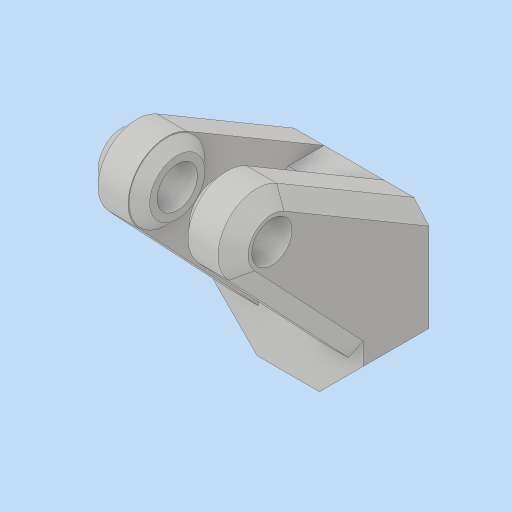
# Autodesk Inventor part: kladka-midwheel_wBearing-atTprofile
Saved by Autodesk Inventor 2024 (Build 280153000, 153)
## iProperties
Created: 2023-04-19
Part Number: kladka-midwheel_wBearing-atTprofile
Material: Generic
Document SubType Name: Modeling
Designer: Karbosch
Density: 1 g/cm^3
Appearance: Default
Mass: 2.94353 g
Surface Area: 19.3732 cm^2
Volume: 2.94353 cm^3
Author: Karbosch
Autodesk Inventor part; units mm, degrees
ref_plane "YZ Plane" through (0, 0, 0) normal (1, 0, 0) x (0, 1, 0)
ref_plane "XZ Plane" through (0, 0, 0) normal (0, 1, 0) x (-1, 0, 0)
ref_plane "XY Plane" through (0, 0, 0) normal (0, 0, 1) x (1, 0, 0)
sketch "Sketch1" plane through (0, 0, 0) normal (0, 0, 1) x (1, 0, 0)
  circle A0 centre (0, 0) radius 2.15
  line L0 (3.3137, 8) -> (8, 3.3137)
  line L1 (8, 3.3137) -> (8, -3.3137)
  line L2 (8, -3.3137) -> (3.3137, -8)
  line L3 (3.3137, -8) -> (-3.3137, -8)
  line L4 (-3.3137, -8) -> (-8, -3.3137)
  line L5 (-8, -3.3137) -> (-8, 3.3137)
  line L6 (-8, 3.3137) -> (-3.3137, 8)
  line L7 (-3.3137, 8) -> (3.3137, 8)
  dimension "d0" = 4.3
  dimension "d1" = 16
  constraints: 16 end point, 2 coincident, 1 centre point, 1 horizontal, 17 other
  measures "d0" diameter of A0
  measures "d1" distance between parallel lines of L3 L7
extrude "Extrusion1" add sketch "Sketch1" along normal blind 7
sketch "Sketch2" plane through (8, -3.3137, 0) normal (1, 0, 0) x (0, 0, -1)
  line L0 (0, 0) -> (-7, 0) projected
  line L1 (0, 6.6274) -> (0, 0) projected
  line L2 (0, 11.3137) -> (0, 6.6274) projected
  circle A0 centre (-16.7618, 16.384) radius 2.15
  circle A1 centre (-16.7618, 16.384) radius 4.15
  line L3 (0, 11.3137) -> (-7, 11.3137) projected
  line L4 (0, 11.3137) -> (-14.6531, 19.9583)
  line L5 (-7, 0) -> (-7, -4.6863) projected
  line L6 (-7, 0) -> (-19.7793, 13.5349)
  line L7 (-7, 1.1637) -> (-7, 5.4637) projected
  line L8 (-7, 3.3137) -> (-11, 3.3137)
  line L9 (-11, 3.3137) -> (-11, 7.0137)
  circle A2 centre (-16.7618, 16.384) radius 11
  point P0 (0, 3.3137)
  dimension "d4" = 4.3
  dimension "d6" = 2
  dimension "d17" = 4
  dimension "d18" = 3.7
  dimension "d19" = 22
  constraints: 8 end point, 4 point on circle, 3 centre point, 2 coincident, 2 tangent, 1 horizontal, 1 midpoint, 1 vertical
  measures "d4" diameter of A0
  measures "d6" radial gap between concentric circles of A1 A0
  measures "d17" distance of L8.start L8.end
  measures "d18" distance of L8.end L9.end
  measures "d19" diameter of A2
extrude "Extrusion2" add sketch "Sketch2" against normal blind 4.8 contours L0 L6 L9 A2 L3 L2 L1 | L3 A2 L4 | L6 A2 L9 | A2 L6 A1 L4 | A1 picked at (-9.3805, 11.8131)
sketch "Sketch4" plane through (0, 0, 7) normal (0, 0, 1) x (1, 0, 0)
  circle A0 centre (0, 0) radius 3.7
  dimension "d14" = 7.4
  constraints: 1 centre point, 1 coincident
  measures "d14" diameter of A0
extrude "Extrusion4" cut sketch "Sketch4" along normal through all
chamfer "Chamfer2" distance 1.6 angle 45 3 edges at (8, 15.6589, 20.0055) (8, 3.4538, 13.3896) (8, 12.3223, 7.3265)
chamfer "Chamfer3" distance 3.2 angle 45 1 edges at (-0.0569, 8, 7)
sketch "Sketch5" plane through (3.2, -3.3137, 0) normal (-1, 0, 0) x (0, 0, 1)
  circle A0 centre (16.7618, 16.384) radius 2.15 projected
  arc A1 (18.6159, 14.6333) -> (15.4661, 18.5803) centre (16.7618, 16.384) ccw projected
  circle A2 centre (16.7618, 16.384) radius 2.95
  point P0 (0, 3.3137)
  dimension "d26" = 0.8
  constraints: 1 centre point, 1 coincident
  measures "d26" radial gap between concentric circles of A0 A2
extrude "Extrusion5" add sketch "Sketch5" along normal blind 1.1
chamfer "Chamfer4" distance 1.1 angle 45 1 edges at (3.2, 13.0703, 13.8118)
mirror "Mirror2" about plane through (0, 0, 0) normal (1, 0, 0) of "Extrusion2", "Extrusion5", "Chamfer4", "Chamfer2"
body "Solid1"
